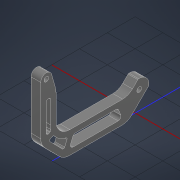
# Autodesk Inventor part: Swing-Arm B
Saved by Autodesk Inventor 2022.2 (Build 262287010, 287A)
## iProperties
Created: 2022-03-22
Part Number: Swing-Arm B
Material: ABS-Kunststoff
Document SubType Name: Modeling
Designer: sleib
Density: 1.06 g/cm^3
Appearance: Glatt - Schwarz
Author: sleib
Autodesk Inventor part; units mm, degrees
ref_plane "YZ Plane" through (0, 0, 0) normal (1, 0, 0) x (0, 1, 0)
ref_plane "XZ Plane" through (0, 0, 0) normal (0, 1, 0) x (-1, 0, 0)
ref_plane "XY Plane" through (0, 0, 0) normal (0, 0, 1) x (1, 0, 0)
sketch "SwingArm A" plane through (0, 0, 0) normal (0, 0, 1) x (1, 0, 0)
  line L0 (-13.1129, 5.4447) -> (-1.1226, -6.6888)
  arc A0 (6.9887, 0.3969) -> (6.7016, 1.0431) centre (5.9903, 0.3402) ccw
  arc A1 (-1.1226, -6.6888) -> (-0.4798, -6.9835) centre (-0.4113, -5.9859) ccw
  line L1 (40, 71) -> (4.8211, 71)
  line L2 (28.3926, 60) -> (0, 60) construction
  line L3 (-2.2079, 68.1129) -> (-13.029, 57.4195)
  line L4 (-16, 50.3066) -> (-16, 12.4737)
  line L5 (0, 60) -> (0, 11.9322) construction
  line L6 (2.8871, 4.9032) -> (6.7016, 1.0431)
  circle A2 centre (0, 0) radius 1.7
  circle A3 centre (40, 67) radius 1.7
  line L7 (40, 67) -> (-8, 67) construction
  line L8 (-8, 67) -> (-8, 8.0955) construction
  line L9 (-8, 8.0955) -> (0, 0) construction
  line L10 (41.0716, 63.1462) -> (31.0716, 60.3655)
  arc A4 (28.3926, 60) -> (31.0716, 60.3655) centre (28.3926, 70) ccw
  circle A5 centre (40, 67) radius 4 construction
  arc A6 (41.0716, 63.1462) -> (40, 71) centre (40, 67) ccw
  circle A7 centre (0, 0) radius 5.5 construction
  arc A8 (10, 60) -> (0, 50) centre (10, 50) ccw
  arc A9 (0, 11.9322) -> (2.8871, 4.9032) centre (10, 11.9322) ccw
  arc A10 (-16, 12.4737) -> (-13.1129, 5.4447) centre (-6, 12.4737) ccw
  arc A11 (-13.029, 57.4195) -> (-16, 50.3066) centre (-6, 50.3066) ccw
  arc A12 (4.8211, 71) -> (-2.2079, 68.1129) centre (4.8211, 61) ccw
  line L11 (-9.2401, 13.305) -> (-5.2401, 14.948)
  line L12 (-4, 16.798) -> (-4, 45.9717)
  line L13 (-5.2292, 47.8172) -> (-9.2292, 49.488)
  line L14 (-12, 47.6425) -> (-12, 15.155)
  arc A13 (-4, 45.9717) -> (-5.2292, 47.8172) centre (-6, 45.9717) ccw
  arc A14 (-9.2292, 49.488) -> (-12, 47.6425) centre (-10, 47.6425) ccw
  arc A15 (-5.2401, 14.948) -> (-4, 16.798) centre (-6, 16.798) ccw
  arc A16 (-12, 15.155) -> (-9.2401, 13.305) centre (-10, 15.155) ccw
  line L15 (28.3926, 60) -> (10, 60)
  line L16 (0, 50) -> (0, 11.9322)
  line L17 (1.3855, 64.1003) -> (2.0531, 62.4749)
  line L18 (-5.0798, 52.0897) -> (-9.0729, 53.7576)
  line L19 (-0.2424, 64.4316) -> (-9.3904, 55.3916)
  arc A17 (1.7195, 61.2887) -> (2.0531, 62.4749) centre (1.1281, 62.095) ccw
  arc A18 (1.3855, 64.1003) -> (-0.2424, 64.4316) centre (0.4605, 63.7204) ccw
  arc A19 (-5.0798, 52.0897) -> (-3.7148, 52.8116) centre (-4.6944, 53.0125) ccw
  arc A20 (-9.3904, 55.3916) -> (-9.0729, 53.7576) centre (-8.6875, 54.6803) ccw
  line L20 (-15.2274, 54.1608) -> (0, 47.8005) construction
  arc A21 (-0.4798, -6.9835) -> (6.9887, 0.3969) centre (0, 0) ccw
  arc A22 (1.7195, 61.2887) -> (-3.7148, 52.8116) centre (10, 50) ccw
  line L21 (0.0419, 2.0916) -> (2.8931, -0.7936) construction
  arc A23 (0.7592, -2.9023) -> (2.8931, -0.7936) centre (0, 0) ccw construction
  line L22 (0.7592, -2.9023) -> (-10.2677, 8.2563) construction
  arc A24 (-12, 12.4737) -> (-10.2677, 8.2563) centre (-6, 12.4737) ccw construction
  line L23 (-12, 12.4737) -> (-12, 50.3066) construction
  arc A25 (-10.2174, 54.5744) -> (-12, 50.3066) centre (-6, 50.3066) ccw construction
  line L24 (-10.2174, 54.5744) -> (0.6037, 65.2677) construction
  arc A26 (4.8211, 67) -> (0.6037, 65.2677) centre (4.8211, 61) ccw construction
  line L25 (4.8211, 67) -> (40, 67) construction
  line L26 (40, 67) -> (30, 64.2193) construction
  arc A27 (28.3926, 64) -> (30, 64.2193) centre (28.3926, 70) ccw construction
  line L27 (28.3926, 64) -> (10, 64) construction
  arc A28 (10, 64) -> (-4, 50) centre (10, 50) ccw construction
  line L28 (-4, 50) -> (-4, 11.9322) construction
  arc A29 (-4, 11.9322) -> (0.0419, 2.0916) centre (10, 11.9322) ccw construction
  line L29 (-15.2501, 8.6743) -> (0, 14.9381) construction
  line L30 (1.0217, 70.2501) -> (5.6423, 59.0006) construction
  line L31 (29.7445, 60.0918) -> (28.2561, 71) construction
  line L32 (5.6582, 64.2257) -> (5.0855, 65.6201)
  line L33 (26.9014, 66.1352) -> (27.0378, 65.1352)
  line L34 (25.9106, 67) -> (6.0106, 67)
  line L35 (26.047, 64) -> (10, 64)
  arc A30 (10, 64) -> (6.811, 63.632) centre (10, 50) ccw
  arc A31 (5.6582, 64.2257) -> (6.811, 63.632) centre (6.5833, 64.6057) ccw
  arc A32 (6.0106, 67) -> (5.0855, 65.6201) centre (6.0106, 66) ccw
  arc A33 (26.9014, 66.1352) -> (25.9106, 67) centre (25.9106, 66) ccw
  arc A34 (26.047, 64) -> (27.0378, 65.1352) centre (26.047, 65) ccw
  point P0 (-12, 31.3902)
  point P1 (-16, 31.3902)
  dimension "d0" = 3.4
  dimension "d1" = 3.4
  dimension "d2" = 7
  dimension "d3" = 4
  dimension "d6" = 10
  dimension "d7" = 16
  dimension "d8" = 67
  dimension "d9" = 10
  dimension "d10" = 10
  dimension "d11" = 10
  dimension "d12" = 10
  dimension "d13" = 10
  dimension "d14" = 40
  dimension "d15" = 134.66
  dimension "d16" = 2
  dimension "d17" = 2
  dimension "d18" = 1
  dimension "d20" = 4
  dimension "d24" = 10
  dimension "d25" = 50
  dimension "d32" = 7
  dimension "d33" = 11
  dimension "d34" = 1
  dimension "d35" = 4
  dimension "d37" = 2
  dimension "d38" = 4
  dimension "d39" = 1
  dimension "d41" = 2
  dimension "d42" = 1
  dimension "d43" = 1
  measures "d0" diameter of A2
  measures "d1" diameter of A3
  measures "d2" distance between parallel lines of L2 L7
  measures "d3" distance between parallel lines of L7 L1
  measures "d6" radius of A4
  measures "d7" distance between parallel lines of L4 L5
  measures "d8" vertical distance of L9.end point (40, 67)
  measures "d9" radius of A8
  measures "d10" radius of A9
  measures "d11" radius of A10
  measures "d12" radius of A12
  measures "d13" radius of A11
  measures "d14" horizontal distance of L9.end L7.start
  measures "d15" angle of L4 L3
  measures "d16" radius of A14
  measures "d17" radius of A13
  measures "d18" radius of A18
  measures "d20" distance between parallel lines of L13 L18
  measures "d24" horizontal distance of L10.start L10.end
  measures "d25" distance from line of L9.end L3
  measures "d32" radius of A21
  measures "d33" diameter of A7
  measures "d34" radius of A0
  measures "d35" radial gap between concentric circles of A9 A29
  measures "d37" distance between parallel lines of L29 L11
  measures "d38" distance between parallel lines of L32 L17
  measures "d39" radius of A32
  measures "d41" distance between parallel lines of L33 L31
  measures "d42" radius of A33
  measures "d43" radius of A20
sketch "Skizze1" plane through (0, 0, 0) normal (1, 0, 0) x (0, 1, 0)
  line L0 (43.1754, 67) -> (41.5877, 64.25)
  line L1 (41.5877, 64.25) -> (38.4123, 64.25)
  line L2 (38.4123, 64.25) -> (36.8246, 67)
  line L3 (36.8246, 67) -> (38.4123, 69.75)
  line L4 (38.4123, 69.75) -> (41.5877, 69.75)
  line L5 (41.5877, 69.75) -> (43.1754, 67)
  line L6 (2.232, -2.2587) -> (-0.84, -3.0623)
  line L7 (-0.84, -3.0623) -> (-3.072, -0.8036)
  line L8 (-3.072, -0.8036) -> (-2.232, 2.2587)
  line L9 (-2.232, 2.2587) -> (0.84, 3.0623)
  line L10 (0.84, 3.0623) -> (3.072, 0.8036)
  line L11 (3.072, 0.8036) -> (2.232, -2.2587)
  line L12 (-13.1129, 5.4447) -> (-1.1226, -6.6888)
  arc A0 (6.9887, 0.3969) -> (6.7016, 1.0431) centre (5.9903, 0.3402) ccw
  arc A1 (-1.1226, -6.6888) -> (-0.4798, -6.9835) centre (-0.4113, -5.9859) ccw
  line L13 (40, 71) -> (4.8211, 71)
  line L14 (28.3926, 60) -> (0, 60) construction
  line L15 (-2.2079, 68.1129) -> (-13.029, 57.4195)
  line L16 (-16, 50.3066) -> (-16, 12.4737)
  line L17 (0, 60) -> (0, 11.9322) construction
  line L18 (2.8871, 4.9032) -> (6.7016, 1.0431)
  circle A2 centre (0, 0) radius 1.7
  circle A3 centre (40, 67) radius 1.7
  line L19 (40, 67) -> (-8, 67) construction
  line L20 (-8, 67) -> (-8, 8.0955) construction
  line L21 (-8, 8.0955) -> (0, 0) construction
  line L22 (41.0716, 63.1462) -> (31.0716, 60.3655)
  arc A4 (28.3926, 60) -> (31.0716, 60.3655) centre (28.3926, 70) ccw
  circle A5 centre (40, 67) radius 4 construction
  arc A6 (41.0716, 63.1462) -> (40, 71) centre (40, 67) ccw
  circle A7 centre (0, 0) radius 5.5 construction
  arc A8 (10, 60) -> (0, 50) centre (10, 50) ccw
  arc A9 (0, 11.9322) -> (2.8871, 4.9032) centre (10, 11.9322) ccw
  arc A10 (-16, 12.4737) -> (-13.1129, 5.4447) centre (-6, 12.4737) ccw
  arc A11 (-13.029, 57.4195) -> (-16, 50.3066) centre (-6, 50.3066) ccw
  arc A12 (4.8211, 71) -> (-2.2079, 68.1129) centre (4.8211, 61) ccw
  line L23 (-9.2401, 13.305) -> (-5.2401, 14.948)
  line L24 (-4, 16.798) -> (-4, 45.9717)
  line L25 (-5.2292, 47.8172) -> (-9.2292, 49.488)
  line L26 (-12, 47.6425) -> (-12, 15.155)
  arc A13 (-4, 45.9717) -> (-5.2292, 47.8172) centre (-6, 45.9717) ccw
  arc A14 (-9.2292, 49.488) -> (-12, 47.6425) centre (-10, 47.6425) ccw
  arc A15 (-5.2401, 14.948) -> (-4, 16.798) centre (-6, 16.798) ccw
  arc A16 (-12, 15.155) -> (-9.2401, 13.305) centre (-10, 15.155) ccw
  line L27 (28.3926, 60) -> (10, 60)
  line L28 (0, 50) -> (0, 11.9322)
  line L29 (1.3855, 64.1003) -> (2.0531, 62.4749)
  line L30 (-5.0798, 52.0897) -> (-9.0729, 53.7576)
  line L31 (-0.2424, 64.4316) -> (-9.3904, 55.3916)
  arc A17 (1.7195, 61.2887) -> (2.0531, 62.4749) centre (1.1281, 62.095) ccw
  arc A18 (1.3855, 64.1003) -> (-0.2424, 64.4316) centre (0.4605, 63.7204) ccw
  arc A19 (-5.0798, 52.0897) -> (-3.7148, 52.8116) centre (-4.6944, 53.0125) ccw
  arc A20 (-9.3904, 55.3916) -> (-9.0729, 53.7576) centre (-8.6875, 54.6803) ccw
  line L32 (-15.2274, 54.1608) -> (0, 47.8005) construction
  arc A21 (-0.4798, -6.9835) -> (6.9887, 0.3969) centre (0, 0) ccw
  arc A22 (1.7195, 61.2887) -> (-3.7148, 52.8116) centre (10, 50) ccw
  line L33 (0.0419, 2.0916) -> (2.8931, -0.7936) construction
  arc A23 (0.7592, -2.9023) -> (2.8931, -0.7936) centre (0, 0) ccw construction
  line L34 (0.7592, -2.9023) -> (-10.2677, 8.2563) construction
  arc A24 (-12, 12.4737) -> (-10.2677, 8.2563) centre (-6, 12.4737) ccw construction
  line L35 (-12, 12.4737) -> (-12, 50.3066) construction
  arc A25 (-10.2174, 54.5744) -> (-12, 50.3066) centre (-6, 50.3066) ccw construction
  line L36 (-10.2174, 54.5744) -> (0.6037, 65.2677) construction
  arc A26 (4.8211, 67) -> (0.6037, 65.2677) centre (4.8211, 61) ccw construction
  line L37 (4.8211, 67) -> (40, 67) construction
  line L38 (40, 67) -> (30, 64.2193) construction
  arc A27 (28.3926, 64) -> (30, 64.2193) centre (28.3926, 70) ccw construction
  line L39 (28.3926, 64) -> (10, 64) construction
  arc A28 (10, 64) -> (-4, 50) centre (10, 50) ccw construction
  line L40 (-4, 50) -> (-4, 11.9322) construction
  arc A29 (-4, 11.9322) -> (0.0419, 2.0916) centre (10, 11.9322) ccw construction
  line L41 (-15.2501, 8.6743) -> (0, 14.9381) construction
  line L42 (1.0217, 70.2501) -> (5.6423, 59.0006) construction
  line L43 (29.7445, 60.0918) -> (28.2561, 71) construction
  line L44 (5.6582, 64.2257) -> (5.0855, 65.6201)
  line L45 (26.9014, 66.1352) -> (27.0378, 65.1352)
  line L46 (25.9106, 67) -> (6.0106, 67)
  line L47 (26.047, 64) -> (10, 64)
  arc A30 (10, 64) -> (6.811, 63.632) centre (10, 50) ccw
  arc A31 (5.6582, 64.2257) -> (6.811, 63.632) centre (6.5833, 64.6057) ccw
  arc A32 (6.0106, 67) -> (5.0855, 65.6201) centre (6.0106, 66) ccw
  arc A33 (26.9014, 66.1352) -> (25.9106, 67) centre (25.9106, 66) ccw
  arc A34 (26.047, 64) -> (27.0378, 65.1352) centre (26.047, 65) ccw
  point P0 (0, 0)
  point P1 (40, 67)
  dimension "d50" = 5.5
  dimension "d51" = 5.5
  constraints: 24 end point, 31 other
  measures "d50" distance between parallel lines of L7 L10
  measures "d51" distance between parallel lines of L1 L4
extrude "Extrusion1" add sketch "Skizze1" along normal blind 3 and the other way blind 4 contours L0 L1 L2 L3 L4 L5 | L6 L7 L8 L9 L10 L11 | A10 L16 A11 L15 A12 L13 A6 L22 A4 L27 A8 L28 A9 L18 A0 A21 A1 L12
extrude "Extrusion2" cut sketch "Skizze1" against normal through all contours L0 L1 L2 L3 L4 L5 | L6 L7 L8 L9 L10 L11
